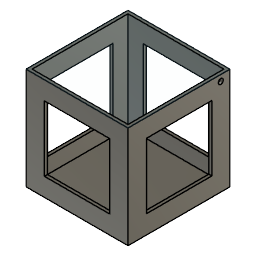
cube_frame (Autodesk Fusion 360 design; units mm, degrees)
part number: 2026-06-15-21-02-12-768
Autodesk Fusion 360 part; units mm, degrees
sketch "Sketch1" plane through (0, 0, 0) normal (0, 0, 1) x (1, 0, 0)
  line L0 (-50, 50) -> (60, 50)
  line L1 (60, 50) -> (60, -50)
  line L2 (60, -50) -> (-50, -50)
  line L3 (-50, -50) -> (-50, 50)
  constraint horizontal L0
  constraint vertical L1
  constraint horizontal L2
  constraint vertical L3
sketch "Sketch8" plane through (0, 0, 0) normal (0, 0, 1) x (1, 0, 0)
  line L0 (-50, 50) -> (50, 50)
  line L1 (50, 50) -> (50, -50)
  line L2 (50, -50) -> (-50, -50)
  line L3 (-50, -50) -> (-50, 50)
  line L4 (-50, 50) -> (50, -50) construction
  line L5 (50, 50) -> (-50, -50) construction
  dimension "d15" = 100
  dimension "d16" = 100
  constraint horizontal L0
  constraint perpendicular L0 L1
  constraint parallel L0 L2
  constraint parallel L1 L3
  constraint coincident L4 origin
  constraint coincident L5 origin
  measures "d15" distance of L0.end L1.end
  measures "d16" distance of L0.start L0.end
extrude "Extrude3" add sketch "Sketch8" along normal blind 100
sketch "Sketch9" plane through (0, 0, 100) normal (0, 0, 1) x (-1, 0, 0)
  line L0 (50, 50) -> (-50, 50)
  line L1 (-50, 50) -> (-50, -50)
  line L2 (-50, -50) -> (50, -50)
  line L3 (50, -50) -> (50, 50)
shell "Shell2" thickness 3 removed faces 1 at (-16.6667, 16.6667, 100)
sketch "Sketch10" plane through (50, 0, 0) normal (1, 0, 0) x (0, 1, 0)
  line L0 (-50, 0) -> (50, 0)
  line L1 (50, 0) -> (50, 100)
  line L2 (50, 100) -> (-50, 100)
  line L3 (-50, 100) -> (-50, 0)
  line L4 (32.2521, 82.1964) -> (-31.7479, 82.1964)
  line L5 (-31.7479, 82.1964) -> (-31.7479, 18.1964)
  line L6 (-31.7479, 18.1964) -> (32.2521, 18.1964)
  line L7 (32.2521, 18.1964) -> (32.2521, 82.1964)
  line L8 (32.2521, 82.1964) -> (-31.7479, 18.1964) construction
  line L9 (-31.7479, 82.1964) -> (32.2521, 18.1964) construction
  point P0 (0.2521, 50.1964)
  dimension "d20" = 64
  dimension "d21" = 64
  constraint horizontal L4
  constraint perpendicular L4 L5
  constraint parallel L4 L6
  constraint parallel L5 L7
  constraint coincident L8 P0
  constraint coincident L9 P0
  measures "d20" distance of L5.end L6.end
  measures "d21" distance of L4.end L5.end
extrude "Extrude4" cut sketch "Sketch10" against normal through all contours L4 L5 L6 L7
sketch "Sketch11" plane through (0, -50, 0) normal (0, -1, 0) x (1, 0, 0)
  line L0 (-50, 0) -> (50, 0)
  line L1 (50, 0) -> (50, 100)
  line L2 (50, 100) -> (-50, 100)
  line L3 (-50, 100) -> (-50, 0)
  line L4 (-32, 82) -> (32, 82)
  line L5 (32, 82) -> (32, 18)
  line L6 (32, 18) -> (-32, 18)
  line L7 (-32, 18) -> (-32, 82)
  line L8 (-32, 82) -> (32, 18) construction
  line L9 (32, 82) -> (-32, 18) construction
  point P0 (0, 50)
  dimension "d23" = 64
  dimension "d24" = 64
  constraint horizontal L4
  constraint perpendicular L4 L5
  constraint parallel L4 L6
  constraint parallel L5 L7
  constraint coincident L8 P0
  constraint coincident L9 P0
  measures "d23" distance of L4.start L4.end
  measures "d24" distance of L4.end L5.end
extrude "Extrude5" cut sketch "Sketch11" against normal blind 110 contours L4 L5 L6 L7
sketch "Sketch12" plane through (0, 0, 0) normal (0, 0, 1) x (1, 0, 0)
  line L0 (35.1289, -20.848) -> (20.1289, -20.848)
  line L1 (20.1289, -20.848) -> (20.1289, -28.848)
  line L2 (20.1289, -28.848) -> (35.1289, -28.848)
  line L3 (35.1289, -28.848) -> (35.1289, -20.848)
  dimension "d27" = 15
  dimension "d28" = 8
  constraint horizontal L0
  constraint vertical L1
  constraint horizontal L2
  constraint vertical L3
  measures "d27" distance of L0.start L0.end
  measures "d28" distance of L0.start L2.end
extrude "Extrude6" cut sketch "Sketch12" along normal blind 3
sketch "Sketch13" plane through (50, 0, 0) normal (1, 0, 0) x (0, 1, 0)
  line L0 (32.2521, 18.1964) -> (-31.7479, 18.1964)
  line L1 (-31.7479, 18.1964) -> (-31.7479, 82.1964)
  line L2 (-31.7479, 82.1964) -> (32.2521, 82.1964)
  line L3 (32.2521, 82.1964) -> (32.2521, 18.1964)
  line L4 (-50, 0) -> (50, 0)
  line L5 (50, 0) -> (50, 100)
  line L6 (50, 100) -> (-50, 100)
  line L7 (-50, 100) -> (-50, 0)
  circle A0 centre (41, 94) radius 2.5
  dimension "d31" = 5
  measures "d31" diameter of A0
extrude "Extrude7" cut sketch "Sketch13" against normal blind 3 contours A0
